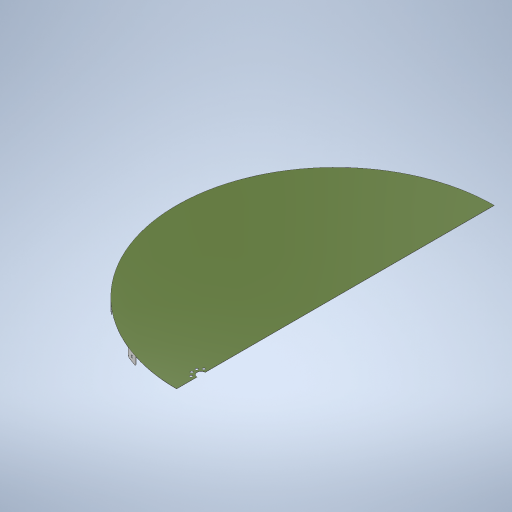
# Autodesk Inventor part: Aspa2_1
Saved by Autodesk Inventor 2024 (Build 280153000, 153)
## iProperties
Created: 2024-04-25
Part Number: Aspa2_1
Material: Genérico
Document SubType Name: Modeling
Designer: alexa
Density: 1 g/cm^3
Appearance: Valor por defecto
Author: alexa
Autodesk Inventor part; units mm, degrees
note: some values were not read from the file. Chosen so that the rebuilt part matches the saved one: pattern direction of "Circular Pattern1".
sketch "Sketch1" plane through (0, 0, 0) normal (0, 1, 0) x (-1, 0, 0)
  arc A0 (0, -194.17) -> (0, 194.17) centre (0, 0) ccw
  line L0 (0, 0) -> (0, 194.17) construction
  line L1 (0, 0) -> (0, -194.17) construction
  line L2 (0, -194.17) -> (0, 194.17)
  line L3 (0, 194.17) -> (0, -194.17)
  dimension "d0" = 194.17
  dimension "d1" = 180
  constraints: 8 end point, 2 point on circle, 1 centre point, 1 coincident
  measures "d0" radius of A0
  measures "d1" angle of L0 L1
extrude "Extrusion1" add sketch "Sketch1" along normal blind 0.27
ref_plane "Work Plane1" through (0, 0, 0) normal (0, -1, 0) x (1, 0, 0)
sketch "Sketch3" plane through (0, 0, 0) normal (0, -1, 0) x (1, 0, 0)
  arc A0 (0, 194.17) -> (0, -194.17) centre (0, 0) ccw projected
  arc A1 (-194.0149, 7.7585) -> (-194.0149, -7.7585) centre (0, 0) ccw
  line L0 (0, 0) -> (-194.0149, 7.7585) construction
  line L1 (0, 0) -> (194.17, 0) construction
  line L2 (0, 0) -> (-194.0149, -7.7585) construction
  arc A2 (-193.7451, 7.7477) -> (-193.7451, -7.7477) centre (0, 0) ccw
  line L3 (0, 0) -> (-193.7451, 7.7477) construction
  line L4 (0, 0) -> (193.9, 0) construction
  line L5 (0, 0) -> (-193.7451, -7.7477) construction
  line L6 (-194.0149, 7.7585) -> (-193.7451, 7.7477)
  line L7 (-194.0149, -7.7585) -> (-193.7451, -7.7477)
  point P0 (-194.0149, -7.7585)
  dimension "d16" = 177.71
  dimension "d17" = 4.58
  dimension "d18" = 193.9
  dimension "d19" = 177.71
  dimension "d20" = 4.58
  constraints: 16 end point, 5 point on circle, 2 centre point, 2 coincident, 2 equal length, 2 horizontal
  measures "d16" angle of L1 L0
  measures "d17" angle of L0 L2
  measures "d18" radius of A2
  measures "d19" angle of L4 L3
  measures "d20" angle of L3 L5
extrude "Extrusion3" add sketch "Sketch3" along normal blind 10
fillet "Fillet3" radius 2 2 edges at (-193.88, -10, 7.7531) (-193.88, -10, -7.7531)
ref_plane "Work Plane2" through (-194.17, 0, 0) normal (1, 0, 0) x (0, 1, 0)
sketch "Sketch4" plane through (-194.17, 0, 0) normal (1, 0, 0) x (0, 1, 0)
  circle A0 centre (-4.7221, 0) radius 1.5
  point P0 (0, 0)
  dimension "d26" = 3
  constraints: 1 centre point
  measures "d26" diameter of A0
extrude "Extrusion4" cut sketch "Sketch4" along normal blind 1
pattern_circular "Circular Pattern1" count 7 over 140 about axis through (0, -10, 0) along (0, 1, 0) of "Extrusion3", "Fillet3", "Extrusion4" both ways yes
ref_plane "Work Plane3" through (0, 0.27, 0) normal (0, 1, 0) x (1, 0, 0)
sketch "Sketch5" plane through (0, 0.27, 0) normal (0, 1, 0) x (1, 0, 0)
  arc A0 (0, 194.17) -> (0, -194.17) centre (0, 0) ccw projected
  line L0 (0, -194.17) -> (0, 194.17) projected
  arc A1 (0, -159.17) -> (0, -169.17) centre (0, -164.17) ccw
  line L1 (0, -164.17) -> (0, -169.17) construction
  line L2 (0, -164.17) -> (0, -159.17) construction
  line L3 (0, -169.17) -> (0, -159.17)
  line L4 (0, -169.17) -> (0, -159.17)
  line L5 (0, -164.17) -> (9, -164.17) construction
  line L6 (0, -164.17) -> (9, -164.17) construction
  circle A2 centre (-4.5, -171.9642) radius 1.5
  circle A3 centre (-8.4572, -167.2482) radius 1.5
  circle A4 centre (-8.4572, -161.0918) radius 1.5
  circle A5 centre (-4.5, -156.3758) radius 1.5
  point P0 (0, -169.17)
  dimension "d34" = 5
  dimension "d35" = 180
  dimension "d43" = 3
  dimension "d46" = 120
  constraints: 12 end point, 5 centre point, 2 horizontal, 2 point on circle, 1 point on line, 1 vertical, 7 other
  measures "d34" radius of A1
  measures "d35" angle of L1 L2
  measures "d43" diameter of A2
extrude "Extrusion5" cut sketch "Sketch5" against normal blind 1 contours L0 A1 | A2 | A3 | A4 | A5
body "Solid1"
